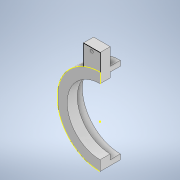
# Autodesk Inventor part: ARMR
Saved by Autodesk Inventor 2022 (Build 260153000, 153)
## iProperties
Created: 2023-03-07
Part Number: ARMR
Material: 一般
Document SubType Name: Modeling
Designer: robot
Density: 1 g/cm^3
Appearance: 預設
Mass: 20.4629 g
Surface Area: 85.019 cm^2
Volume: 20.4629 cm^3
Author: robot
Autodesk Inventor part; units mm, degrees
ref_plane "YZ Plane" through (0, 0, 0) normal (1, 0, 0) x (0, 1, 0)
ref_plane "XZ Plane" through (0, 0, 0) normal (0, 1, 0) x (-1, 0, 0)
ref_plane "XY Plane" through (0, 0, 0) normal (0, 0, 1) x (1, 0, 0)
sketch "草圖1" plane through (0, 0, 0) normal (0, 0, 1) x (1, 0, 0)
  arc A0 (0, 32.5) -> (0, -32.5) centre (0, 0) ccw
  arc A1 (0, 37.5) -> (0, -37.5) centre (0, 0) ccw
  arc A2 (0, 42.5) -> (0, -42.5) centre (0, 0) ccw
  line L0 (0, 0) -> (0, -59.8463)
  line L1 (0, -59.8463) -> (0, 72.1748)
  point P0 (0, -37.5)
  point P1 (0, -42.5)
  dimension "d16" = 32.5
  dimension "d17" = 37.5
  dimension "d18" = 42.5
  constraints: 7 point on line, 6 point on circle, 4 end point, 3 centre point, 3 coincident, 1 vertical
  measures "d16" radius of A0
  measures "d17" radius of A1
  measures "d18" radius of A2
extrude "擠出1" add sketch "草圖1" along normal blind 10 contours A0 L0 A1 L1
extrude "擠出2" add sketch "草圖1" along normal mid plane 20 contours A1 L0 A2 L1
sketch "草圖2" plane through (0, 0, 10) normal (0, 0, 1) x (1, 0, 0)
  line L0 (0, 32.5) -> (0, 42.5) projected
  line L1 (0, 42.5) -> (0, 52.5)
  arc A0 (0, 42.5) -> (0, -42.5) centre (0, 0) ccw projected
  line L2 (-16.411, 39.2037) -> (-16.411, 59.2037)
  line L3 (-16.411, 59.2037) -> (0, 59.2037)
  line L4 (0, 59.2037) -> (0, 42.5)
  dimension "d4" = 10
  dimension "d9" = 20
  dimension "d13" = 16.411
  constraints: 8 end point, 2 vertical, 1 horizontal, 1 perpendicular, 1 point on circle
  measures "d4" distance of L0.end L1.end
  measures "d9" distance of L2.start L2.end
  measures "d13" distance of L2.end L3.end
extrude "擠出3" add sketch "草圖2" against normal blind 10
sketch "草圖4" plane through (0, 0, 10) normal (0, 0, 1) x (1, 0, 0)
  line L0 (0, 59.2037) -> (0, 37.5) projected
  line L1 (-16.411, 59.2037) -> (-16.411, 39.2037) projected
  line L2 (-16.411, 59.2037) -> (-8.206, 59.2037)
  line L3 (-8.206, 59.2037) -> (-8.206, 56.2037)
  circle A0 centre (-8.206, 56.2037) radius 1.5
  point P0 (0, 0)
  dimension "d21" = 8.205
  dimension "d22" = 3
  dimension "d23" = 3
  constraints: 4 end point, 1 centre point, 1 coincident, 1 vertical
  measures "d21" distance of L1.start L2.end
  measures "d22" distance of L2.end L3.end
  measures "d23" diameter of A0
extrude "擠出4" cut sketch "草圖4" against normal blind 20
sketch "草圖5" plane through (0, 0, 10) normal (0, 0, 1) x (1, 0, 0)
  line L0 (-54.3449, 0) -> (9.0575, 0) construction
  line L1 (0, -52.5) -> (0, 52.5) construction
  line L2 (-45.2874, 15) -> (-41, 15)
  line L3 (-41, 15) -> (-41, -15)
  line L4 (-41, -15) -> (-45.2874, -15)
  line L5 (-45.2874, -15) -> (-45.2874, 15)
  point P0 (0, 0)
  dimension "d24" = 15
  dimension "d25" = 15
  dimension "d26" = 41
  constraints: 8 end point, 2 parallel, 1 horizontal, 1 perpendicular
  measures "d24" distance between parallel lines of L0 L2
  measures "d25" distance between parallel lines of L4 L0
  measures "d26" distance between parallel lines of L1 L3
extrude "擠出5" cut sketch "草圖5" against normal blind 28
